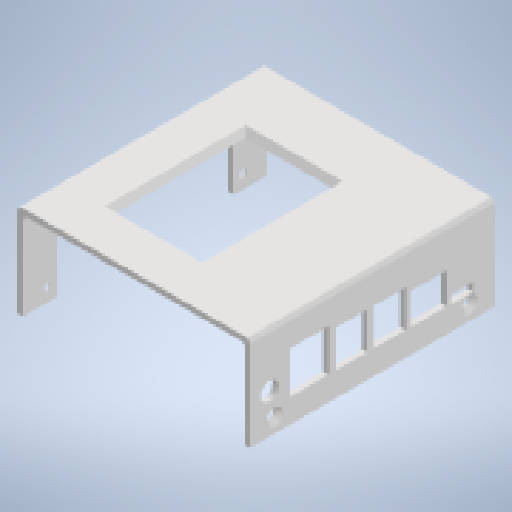
# Autodesk Inventor part: Shroud Top
Saved by Autodesk Inventor 2024 (Build 280153000, 153)
## iProperties
Created: 2023-06-27
Part Number: Shroud Top
Material: Generic
Document SubType Name: Modeling
Designer: TEST BENCH
Density: 1 g/cm^3
Appearance: Default
Author: TEST BENCH
Autodesk Inventor part; units mm, degrees
ref_plane "YZ Plane" through (0, 0, 0) normal (1, 0, 0) x (0, 1, 0)
sketch "Sketch1" plane through (0, 0, 0) normal (0, 0, 1) x (1, 0, 0)
  line L0 (47.5, 19.63) -> (-47.5, 19.63) projected
  arc A0 (-47.5, 19.63) -> (-49.5, 17.63) centre (-47.5, 17.63) ccw projected
  line L1 (-49.5, 17.63) -> (-49.5, -19.63) projected
  line L2 (49.5, -19.63) -> (49.5, 17.63) projected
  arc A1 (49.5, 17.63) -> (47.5, 19.63) centre (47.5, 17.63) ccw projected
  line L3 (-49.5, -19.63) -> (-52, -19.63)
  line L4 (-52, -19.63) -> (-52, 20.13)
  line L5 (-50, 22.13) -> (50, 22.13)
  line L6 (52, 20.13) -> (52, -19.63)
  line L7 (52, -19.63) -> (49.5, -19.63)
  arc A2 (-50, 22.13) -> (-52, 20.13) centre (-50, 20.13) ccw
  arc A3 (52, 20.13) -> (50, 22.13) centre (50, 20.13) ccw
  dimension "d0" = 2.5
  dimension "d1" = 2.5
  dimension "d2" = 2.5
  dimension "d3" = 2
  constraints: 10 end point, 4 point on circle, 4 tangent, 3 perpendicular, 2 centre point, 1 equal radius, 1 horizontal, 1 point on line
  measures "d0" distance between parallel lines of L4 L1
  measures "d1" distance between parallel lines of L2 L6
  measures "d2" distance between parallel lines of L0 L5
  measures "d3" radius of A2
ref_plane "Work Plane1" through (-49.5, -19.63, -109) normal (0, 0, -1) x (0, 1, 0)
extrude "Extrusion1" add sketch "Sketch1" against normal up to surface (109 mm away)
sketch "Sketch2" plane through (-50, 22.13, 0) normal (0, 1, 0) x (1, 0, 0)
  circle A0 centre (39.65, 50.5) radius 18.5 construction
  line L0 (58.85, 79.4) -> (20.45, 79.4) construction
  line L1 (20.45, 79.4) -> (20.45, 21.6) construction
  line L2 (58.85, 21.6) -> (58.85, 79.4) construction
  line L3 (20.45, 21.6) -> (58.85, 21.6) construction
  line L4 (20.15, 23.6) -> (20.15, 77.4) construction
  line L5 (59.15, 77.4) -> (59.15, 23.6) construction
  line L6 (20.15, 21.6) -> (59.15, 21.6) construction
  line L7 (59.15, 79.4) -> (20.15, 79.4) construction
  line L8 (20.15, 21.6) -> (59.15, 21.6)
  line L9 (59.15, 21.6) -> (59.15, 79.4)
  line L10 (59.15, 79.4) -> (20.15, 79.4)
  line L11 (20.15, 79.4) -> (20.15, 21.6)
  line L12 (59.65, 79.4) -> (19.65, 79.4)
  line L13 (19.65, 79.4) -> (19.65, 21.6)
  line L14 (19.65, 21.6) -> (59.65, 21.6)
  line L15 (59.65, 21.6) -> (59.65, 79.4)
  point P0 (50, 0)
  point P1 (59.65, 50.5)
  point P2 (59.15, 79.4)
  dimension "d43" = 40
  dimension "d44" = 39
  dimension "d45" = 0.5
  constraints: 32 end point, 6 horizontal, 4 parallel, 4 vertical, 2 perpendicular, 1 midpoint, 12 other
  measures "d43" distance from line of L13 point (59.65, 50.5)
  measures "d44" distance between parallel lines of L4 L5
  measures "d45" distance between parallel lines of L4 L13
extrude "Extrusion2" cut sketch "Sketch2" against normal up to surface (2.5 mm away)
chamfer "Chamfer1" distance 2.5 angle 45 4 edges at (-10.35, 22.13, -79.4) (-30.35, 22.13, -50.5) (9.65, 22.13, -50.5) (-10.35, 22.13, -21.6)
sketch "Sketch3" plane through (-52, -19.63, 0) normal (-1, 0, 0) x (0, 0, 1)
  line L0 (-94, 9.5) -> (-94, 37.26) projected
  arc A0 (-92, 39.26) -> (-94, 37.26) centre (-92, 37.26) ccw projected
  line L1 (-92, 39.26) -> (-17, 39.26) projected
  arc A1 (-15, 37.26) -> (-17, 39.26) centre (-17, 37.26) ccw projected
  line L2 (-15, 37.26) -> (-15, 9.5) projected
  line L3 (-94, 9.5) -> (-94, 0)
  line L4 (0, 0) -> (-109, 0) construction
  line L5 (-15, 9.5) -> (-15, 0)
  line L6 (-94, 0) -> (-15, 0)
  circle A2 centre (-98, 6.25) radius 1.5 construction
  circle A3 centre (-11, 6.25) radius 1.5 construction
  circle A4 centre (-98, 6.25) radius 1.75
  circle A5 centre (-11, 6.25) radius 1.75
  point P0 (0, 19.63)
  dimension "d13" = 3.5
  dimension "d14" = 3.5
  constraints: 6 end point, 4 centre point, 2 coincident, 2 point on line, 1 collinear, 1 parallel, 1 vertical, 4 other
  measures "d13" diameter of A4
  measures "d14" diameter of A5
ref_plane "Work Plane2" through (-47.0185, 3.2145, -3.5) normal (1, 0, 0) x (0, 1, 0)
extrude "Extrusion3" cut sketch "Sketch3" against normal up to surface (4.9815 mm away)
sketch "Sketch4" plane through (52, -19.63, 0) normal (1, 0, 0) x (0, 0, -1)
  circle A0 centre (98, 6.25) radius 1.5 construction
  circle A1 centre (11, 6.25) radius 1.5 construction
  arc A2 (72.9, 14.47) -> (72.9168, 14.38) centre (73.1508, 14.4702) ccw construction
  line L0 (72.9, 16.76) -> (72.9, 14.47) construction
  line L1 (72.9, 16.76) -> (72.9, 18.76) construction
  line L2 (72.9, 22.14) -> (72.9, 18.76) construction
  arc A3 (73.15, 22.39) -> (72.9, 22.14) centre (73.15, 22.14) ccw construction
  line L3 (73.15, 22.39) -> (85.55, 22.39) construction
  arc A4 (85.8, 22.14) -> (85.55, 22.39) centre (85.55, 22.14) ccw construction
  line L4 (85.8, 22.14) -> (85.8, 18.76) construction
  line L5 (85.8, 18.76) -> (85.8, 16.76) construction
  line L6 (85.8, 16.76) -> (85.8, 14.47) construction
  arc A5 (85.7832, 14.38) -> (85.8, 14.47) centre (85.5492, 14.4702) ccw construction
  line L7 (85.7832, 14.38) -> (86.5, 14.38) construction
  line L8 (86.5, 14.38) -> (86.5, 12.03) construction
  line L9 (81.88, 12.03) -> (86.5, 12.03) construction
  line L10 (81.88, 12.03) -> (81.88, 11.42) construction
  line L11 (81.88, 11.42) -> (86.45, 11.42) construction
  line L12 (87.2, 11.42) -> (86.45, 11.42) construction
  line L13 (87.2, 24.47) -> (87.2, 11.42) construction
  line L14 (87.2, 24.52) -> (87.2, 24.47) construction
  line L15 (87.2, 24.52) -> (71.7, 24.52) construction
  line L16 (71.7, 24.52) -> (71.7, 24.47) construction
  line L17 (71.7, 24.47) -> (71.7, 11.42) construction
  line L18 (71.7, 11.42) -> (72.45, 11.42) construction
  line L19 (72.45, 11.42) -> (76.82, 11.42) construction
  line L20 (76.82, 12.03) -> (76.82, 11.42) construction
  line L21 (72.3, 12.03) -> (76.82, 12.03) construction
  line L22 (72.3, 14.38) -> (72.3, 12.03) construction
  line L23 (72.3, 14.38) -> (72.9168, 14.38) construction
  line L24 (68.675, 20.9412) -> (68.975, 20.9412) construction
  line L25 (68.975, 20.9412) -> (68.975, 26.4362) construction
  arc A6 (68.975, 26.4362) -> (68.375, 27.0362) centre (68.375, 26.4362) ccw construction
  line L26 (68.375, 27.0362) -> (55.825, 27.0362) construction
  arc A7 (55.825, 27.0362) -> (55.225, 26.4362) centre (55.825, 26.4362) ccw construction
  line L27 (55.225, 26.4362) -> (55.225, 20.9412) construction
  line L28 (55.225, 20.9412) -> (55.525, 20.9412) construction
  line L29 (55.525, 26.4362) -> (55.525, 20.9412) construction
  arc A8 (55.825, 26.7362) -> (55.525, 26.4362) centre (55.825, 26.4362) ccw construction
  line L30 (68.375, 26.7362) -> (55.825, 26.7362) construction
  arc A9 (68.675, 26.4362) -> (68.375, 26.7362) centre (68.375, 26.4362) ccw construction
  line L31 (68.675, 26.4362) -> (68.675, 20.9412) construction
  line L32 (51.675, 20.9412) -> (51.975, 20.9412) construction
  line L33 (51.975, 20.9412) -> (51.975, 26.4362) construction
  arc A10 (51.975, 26.4362) -> (51.375, 27.0362) centre (51.375, 26.4362) ccw construction
  line L34 (51.375, 27.0362) -> (38.825, 27.0362) construction
  arc A11 (38.825, 27.0362) -> (38.225, 26.4362) centre (38.825, 26.4362) ccw construction
  line L35 (38.225, 26.4362) -> (38.225, 20.9412) construction
  line L36 (38.225, 20.9412) -> (38.525, 20.9412) construction
  line L37 (38.525, 26.4362) -> (38.525, 20.9412) construction
  arc A12 (38.825, 26.7362) -> (38.525, 26.4362) centre (38.825, 26.4362) ccw construction
  line L38 (51.375, 26.7362) -> (38.825, 26.7362) construction
  arc A13 (51.675, 26.4362) -> (51.375, 26.7362) centre (51.375, 26.4362) ccw construction
  line L39 (51.675, 26.4362) -> (51.675, 20.9412) construction
  line L40 (34.7, 28.373) -> (34.7, 24.4594) construction
  line L41 (30.79, 29.2462) -> (33.9, 29.2462) construction
  line L42 (18.6, 29.2462) -> (21.71, 29.2462) construction
  line L43 (17.8, 25.8062) -> (17.8, 28.4462) construction
  line L44 (17.8, 12.6412) -> (17.8, 25.8412) construction
  line L45 (34.7, 12.6412) -> (34.7, 24.4412) construction
  line L46 (3.1, 11.07) -> (101.9, 11.07) construction
  circle A14 centre (8.5, 17.57) radius 4
  circle A15 centre (11, 6.25) radius 1.75
  circle A16 centre (98, 6.25) radius 1.75
  line L47 (17.55, 29.4962) -> (34.95, 29.4962)
  line L48 (34.95, 29.4962) -> (34.95, 10.82)
  line L49 (34.95, 10.82) -> (17.55, 10.82)
  line L50 (17.55, 10.82) -> (17.55, 29.4962)
  line L51 (37.975, 27.2862) -> (52.225, 27.2862)
  line L52 (52.225, 27.2862) -> (52.225, 10.82)
  line L53 (52.225, 10.82) -> (37.975, 10.82)
  line L54 (37.975, 10.82) -> (37.975, 27.2862)
  line L55 (54.975, 27.2862) -> (69.225, 27.2862)
  line L56 (69.225, 27.2862) -> (69.225, 10.82)
  line L57 (69.225, 10.82) -> (54.975, 10.82)
  line L58 (54.975, 10.82) -> (54.975, 27.2862)
  line L59 (71.45, 24.72) -> (87.45, 24.72)
  line L60 (87.45, 24.72) -> (87.45, 10.82)
  line L61 (87.45, 10.82) -> (71.45, 10.82)
  line L62 (71.45, 10.82) -> (71.45, 24.72)
  line L63 (90.5, 13.2962) -> (90.5, 12.7462) construction
  line L64 (91.35, 13.7962) -> (91, 13.7962) construction
  line L65 (98, 13.7962) -> (97.6, 13.7962) construction
  line L66 (98.5, 13.2962) -> (98.5, 12.7462) construction
  line L67 (89.75, 14.2962) -> (99.25, 14.2962)
  line L68 (99.25, 14.2962) -> (99.25, 10.57)
  line L69 (99.25, 10.57) -> (89.75, 10.57)
  line L70 (89.75, 10.57) -> (89.75, 14.2962)
  line L71 (71.7, 24.47) -> (87.2, 24.47) construction
  line L72 (87.2, 24.47) -> (87.2, 11.07) construction
  line L73 (87.2, 11.07) -> (71.7, 11.07) construction
  line L74 (71.7, 11.07) -> (71.7, 24.47) construction
  circle A17 centre (8.5, 17.57) radius 3.2 projected
  point P0 (0, 19.63)
  point P1 (17.8, 27.1262)
  point P2 (68.975, 23.6887)
  point P3 (91.175, 13.7962)
  point P4 (90.5, 13.0212)
  point P5 (98.5, 13.0212)
  dimension "d15" = 8
  dimension "d16" = 3.5
  dimension "d17" = 3.5
  dimension "d18" = 0.25
  dimension "d19" = 0.25
  dimension "d20" = 0.25
  dimension "d21" = 0.25
  dimension "d22" = 0.25
  dimension "d23" = 0.25
  dimension "d24" = 0.25
  dimension "d25" = 0.25
  dimension "d26" = 0.25
  dimension "d27" = 0.25
  dimension "d28" = 0.25
  dimension "d29" = 0.25
  dimension "d30" = 0.25
  dimension "d31" = 0.25
  dimension "d32" = 0.25
  dimension "d33" = 0.25
  dimension "d34" = 0.5
  dimension "d35" = 0.5
  dimension "d36" = 0.75
  dimension "d37" = 0.75
  constraints: 48 end point, 12 parallel, 6 horizontal, 6 perpendicular, 5 midpoint, 3 centre point, 2 coincident, 2 point on line
  measures "d15" diameter of A14
  measures "d16" diameter of A16
  measures "d17" diameter of A15
  measures "d18" distance between parallel lines of L42 L47
  measures "d19" distance from line of L50 point (17.8, 27.126)
  measures "d20" distance between parallel lines of L48 L40
  measures "d21" distance between parallel lines of L46 L49
  measures "d22" distance between parallel lines of L35 L54
  measures "d23" distance between parallel lines of L34 L51
  measures "d24" distance between parallel lines of L33 L52
  measures "d25" distance between parallel lines of L46 L53
  measures "d26" distance between parallel lines of L26 L55
  measures "d27" distance from line of point (68.975, 23.689) L56
  measures "d28" distance between parallel lines of L27 L58
  measures "d29" distance between parallel lines of L46 L57
  measures "d30" distance between parallel lines of L46 L61
  measures "d31" distance between parallel lines of L59 L71
  measures "d32" distance between parallel lines of L62 L74
  measures "d33" distance between parallel lines of L60 L72
  measures "d34" distance between parallel lines of L46 L69
  measures "d35" distance from line of point (91.175, 13.796) L67
  measures "d36" distance from line of point (90.5, 13.021) L70
  measures "d37" distance from line of point (98.5, 13.021) L68
extrude "Extrusion4" cut sketch "Sketch4" against normal up to surface (2.5 mm away) contours A14 | A15 | A16 | L47 L48 L49 L50 | L51 L52 L53 L54 | L55 L56 L57 L58 | L59 L60 L61 L62 | L67 L68 L69 L70 | A17
chamfer "Chamfer2" distance 2 angle 45 4 edges at (52, -13.38, -9.25) (52, -13.38, -96.25) (-52, -13.38, -99.75) (-52, -13.38, -12.75)
equation "\"d1\" = d0"
equation "\"d2\" = d0"
equation "\"d45\" = -0.5 * d44 + 0.5 * d43"
equation "\"d14\" = d13"
equation "\"d17\" = d16"
equation "\"d19\" = d18"
equation "\"d20\" = d18"
equation "\"d21\" = d18"
equation "\"d22\" = d19"
equation "\"d23\" = d20"
equation "\"d24\" = d23"
equation "\"d25\" = d24"
equation "\"d26\" = d24"
equation "\"d27\" = d26"
equation "\"d28\" = d26"
equation "\"d29\" = d25"
equation "\"d30\" = d29"
equation "\"d31\" = d27"
equation "\"d32\" = d31"
equation "\"d33\" = d31"
equation "\"d34\" = d35"
equation "\"d37\" = d36"
body "Solid1"
